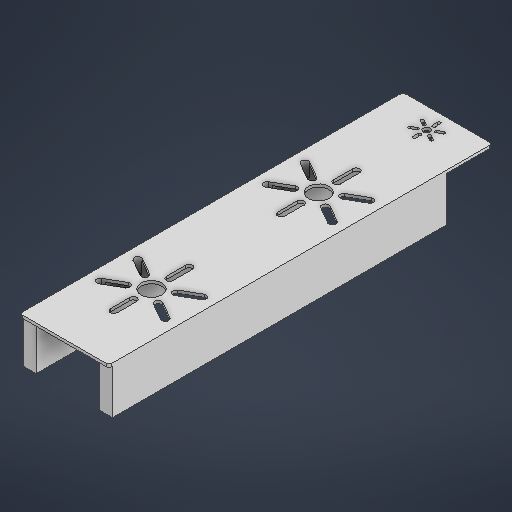
# Autodesk Inventor part: top
Saved by Autodesk Inventor 2027 (Build 310192060, 192F)
## iProperties
Created: 2026-08-21
Part Number: top
Material: Ogólny
Document SubType Name: Modeling
Designer: User
Density: 1 g/cm^3
Appearance: Domyślna
Author: User
Autodesk Inventor part; units mm, degrees
ref_plane "YZ Plane" through (0, 0, 0) normal (1, 0, 0) x (0, 1, 0)
ref_plane "XZ Plane" through (0, 0, 0) normal (0, 1, 0) x (-1, 0, 0)
ref_plane "XY Plane" through (0, 0, 0) normal (0, 0, 1) x (1, 0, 0)
sketch "Szkic1" plane through (0, 0, 0) normal (0, 1, 0) x (-1, 0, 0)
  line L0 (22.75, 95) -> (-22.75, 95)
  line L1 (-22.75, 95) -> (-22.75, -95)
  line L2 (-22.75, -95) -> (22.75, -95)
  line L3 (22.75, -95) -> (22.75, 95)
  line L4 (22.75, 95) -> (-22.75, -95) construction
  line L5 (-22.75, 95) -> (22.75, -95) construction
  line L6 (-32, -97.5) -> (32, -97.5)
  line L7 (32, -97.5) -> (32, 97.5)
  line L8 (32, 97.5) -> (-32, 97.5)
  line L9 (-32, 97.5) -> (-32, -97.5)
  line L10 (-32, -97.5) -> (32, 97.5) construction
  line L11 (32, -97.5) -> (-32, 97.5) construction
  line L12 (32, 97.5) -> (-32, 97.5)
  line L13 (-32, 97.5) -> (-32, 147.5)
  line L14 (-32, 147.5) -> (32, 147.5)
  line L15 (32, 147.5) -> (32, 97.5)
  line L16 (22.75, -95) -> (22.75, -97.5)
  line L17 (-22.75, -95) -> (-22.75, -97.5)
  line L18 (22.75, 95) -> (22.75, 145)
  line L19 (22.75, 145) -> (-22.75, 145)
  line L20 (-22.75, 145) -> (-22.75, 95)
  line L21 (22.75, 145) -> (22.75, 147.5)
  line L22 (-22.75, 145) -> (-22.75, 147.5)
  line L23 (22.75, -95) -> (32, -95)
  line L24 (-22.75, -95) -> (-32, -95)
  line L25 (22.75, 145) -> (32, 145)
  line L26 (-22.75, 145) -> (-32, 145)
  point P0 (0, 0)
  point P1 (0, 0)
  dimension "d0" = 45.5
  dimension "d1" = 190
  dimension "d2" = 64
  dimension "d3" = 195
  dimension "d4" = 50
  dimension "d5" = 50
  dimension "d6" = 0
  dimension "d7" = 0
  constraints: 54 end point, 12 perpendicular, 10 point on line, 6 parallel, 4 midpoint, 2 collinear, 2 horizontal
  measures "d0" distance of L2.end L1.end
  measures "d1" distance of L1.end L0.end
  measures "d2" distance of L9.start L7.end
  measures "d3" distance of L7.end L7.start
  measures "d4" distance of L9.start L14.start
  measures "d5" distance of L0.start L18.end
  measures "d6" distance of point (0, 0) point (0, 0)
  measures "d7" distance of point (0, 0) point (0, 0)
extrude "Wyciągnięcie proste1" add sketch "Szkic1" along normal blind 2
extrude "Wyciągnięcie proste2" add sketch "Szkic1" against normal blind 32 contours L18 L8 L7 L23 L3 | L1 L24 L9 L8 L20 | L18 L25 L15 L8 | L8 L13 L26 L20
sketch "Szkic2" plane through (0, -32, 0) normal (0, -1, 0) x (1, 0, 0)
  line L0 (32, 147.5) -> (-32, 147.5)
  line L1 (-32, -97.5) -> (32, -97.5)
  line L2 (-32, 147.5) -> (32, 147.5)
  line L3 (32, 147.5) -> (32, -97.5)
  line L4 (32, -97.5) -> (-32, -97.5)
  line L5 (-32, -97.5) -> (-32, 147.5)
  line L6 (-32, 147.5) -> (32, 147.5)
  line L7 (0, 147.5) -> (0, -97.5) construction
  line L8 (32, 145) -> (32, -95)
  line L9 (32, -97.5) -> (32, 145)
  line L10 (32, 145) -> (32, 23.75)
  line L11 (32, 23.75) -> (-32, 23.75) construction
  line L12 (22.75, 97.5) -> (22.75, 145)
  line L13 (22.75, 145) -> (22.75, -97.5)
  line L14 (22.75, 23.75) -> (32, 23.75) construction
  line L15 (22.75, 145) -> (22.75, 147.5) construction
  line L16 (22.75, 147.5) -> (32, 147.5) construction
  line L17 (27.375, 147.5) -> (27.375, 23.75) construction
  line L18 (27.375, 147.5) -> (27.375, 137.5) construction
  circle A0 centre (27.375, 137.5) radius 2.4
  circle A1 centre (27.375, 137.5) radius 1
  circle A2 centre (-27.375, 137.5) radius 1
  circle A3 centre (-27.375, 137.5) radius 2.4
  circle A4 centre (-27.375, -90) radius 2.4
  circle A5 centre (-27.375, -90) radius 1
  circle A6 centre (27.375, -90) radius 1
  circle A7 centre (27.375, -90) radius 2.4
  line L19 (-32, -97.5) -> (-32, 147.5) projected
  line L20 (-32, 147.5) -> (32, 147.5)
  point P0 (0, 0)
  point P1 (0, 0)
  dimension "d12" = 10
  dimension "d13" = 4.8
  dimension "d14" = 2
  constraints: 40 end point, 8 centre point, 6 midpoint, 6 symmetric about line, 5 coincident, 4 point on line, 3 collinear, 3 parallel, 3 perpendicular, 1 horizontal, 1 vertical, 6 other
  measures "d12" distance of L17.start L18.end
  measures "d13" diameter of A0
  measures "d14" diameter of A1
extrude "Wyciągnięcie proste3" cut sketch "Szkic2" against normal blind 10 contours A0 | A1 | A2 | A3 | A4 | A5 | A6 | A7
fillet "Zaokrąglenie1" radius 2 2 edges at (32, 1, 147.5) (-32, 1, 147.5)
sketch "Szkic3" plane through (0, 2, 0) normal (0, 1, 0) x (1, 0, 0)
  line L0 (32, 97.5) -> (-32, 97.5) projected
  line L1 (-30, -147.5) -> (30, -147.5) projected
  line L2 (-30, 97.5) -> (30, 97.5)
  line L3 (30, 97.5) -> (30, -147.5)
  line L4 (30, -147.5) -> (-30, -147.5)
  line L5 (-30, -147.5) -> (-30, 97.5)
  line L6 (0, 97.5) -> (0, -147.5) construction
  line L7 (-30, -25) -> (30, -25) construction
  line L8 (0, -25) -> (0, 95) construction
  circle A0 centre (0, 35) radius 7.5
  line L9 (0, 35) -> (0, 55) construction
  line L10 (0, 62) -> (0, 48) construction
  line L11 (-2.5, 62) -> (-2.5, 48)
  line L12 (2.5, 48) -> (2.5, 62)
  arc A1 (2.5, 62) -> (-2.5, 62) centre (0, 62) ccw
  arc A2 (-2.5, 48) -> (2.5, 48) centre (0, 48) ccw
  arc A3 (-12.5083, 39.3349) -> (-10.0083, 43.6651) centre (-11.2583, 41.5) ccw
  line L13 (0, 35) -> (-17.3205, 45) construction
  line L14 (51.9615, 5) -> (-51.9615, 65) construction
  line L15 (-23.3827, 48.5) -> (-11.2583, 41.5) construction
  line L16 (-24.6327, 46.3349) -> (-12.5083, 39.3349)
  line L17 (-10.0083, 43.6651) -> (-22.1327, 50.6651)
  arc A4 (-22.1327, 50.6651) -> (-24.6327, 46.3349) centre (-23.3827, 48.5) ccw
  arc A5 (-10.0083, 26.3349) -> (-12.5083, 30.6651) centre (-11.2583, 28.5) ccw
  line L18 (0, 35) -> (-17.3205, 25) construction
  line L19 (51.9615, 65) -> (-51.9615, 5) construction
  line L20 (-23.3827, 21.5) -> (-11.2583, 28.5) construction
  line L21 (-22.1327, 19.3349) -> (-10.0083, 26.3349)
  line L22 (-12.5083, 30.6651) -> (-24.6327, 23.6651)
  arc A6 (-24.6327, 23.6651) -> (-22.1327, 19.3349) centre (-23.3827, 21.5) ccw
  arc A7 (2.5, 22) -> (-2.5, 22) centre (0, 22) ccw
  line L23 (0, 35) -> (0, 15) construction
  line L24 (0, 95) -> (0, -25) construction
  line L25 (0, 8) -> (0, 22) construction
  line L26 (2.5, 8) -> (2.5, 22)
  line L27 (-2.5, 22) -> (-2.5, 8)
  arc A8 (-2.5, 8) -> (2.5, 8) centre (0, 8) ccw
  arc A9 (12.5083, 30.6651) -> (10.0083, 26.3349) centre (11.2583, 28.5) ccw
  line L28 (0, 35) -> (17.3205, 25) construction
  line L29 (-51.9615, 65) -> (51.9615, 5) construction
  line L30 (23.3827, 21.5) -> (11.2583, 28.5) construction
  line L31 (24.6327, 23.6651) -> (12.5083, 30.6651)
  line L32 (10.0083, 26.3349) -> (22.1327, 19.3349)
  arc A10 (22.1327, 19.3349) -> (24.6327, 23.6651) centre (23.3827, 21.5) ccw
  arc A11 (10.0083, 43.6651) -> (12.5083, 39.3349) centre (11.2583, 41.5) ccw
  line L33 (0, 35) -> (17.3205, 45) construction
  line L34 (-51.9615, 5) -> (51.9615, 65) construction
  line L35 (23.3827, 48.5) -> (11.2583, 41.5) construction
  line L36 (22.1327, 50.6651) -> (10.0083, 43.6651)
  line L37 (12.5083, 39.3349) -> (24.6327, 46.3349)
  arc A12 (24.6327, 46.3349) -> (22.1327, 50.6651) centre (23.3827, 48.5) ccw
  line L38 (0, -147.5) -> (0, 97.5) construction
  line L39 (0, -25) -> (0, -145) construction
  circle A13 centre (0, -85) radius 7.5
  line L40 (0, -85) -> (0, -105) construction
  line L41 (0, -112) -> (0, -98) construction
  line L42 (-2.5, -112) -> (-2.5, -98)
  line L43 (2.5, -98) -> (2.5, -112)
  arc A14 (-2.5, -112) -> (2.5, -112) centre (0, -112) ccw
  arc A15 (2.5, -98) -> (-2.5, -98) centre (0, -98) ccw
  arc A16 (-10.0083, -93.6651) -> (-12.5083, -89.3349) centre (-11.2583, -91.5) ccw
  line L44 (0, -85) -> (-17.3205, -95) construction
  line L45 (51.9615, -55) -> (-51.9615, -115) construction
  line L46 (-23.3827, -98.5) -> (-11.2583, -91.5) construction
  line L47 (-24.6327, -96.3349) -> (-12.5083, -89.3349)
  line L48 (-10.0083, -93.6651) -> (-22.1327, -100.6651)
  arc A17 (-24.6327, -96.3349) -> (-22.1327, -100.6651) centre (-23.3827, -98.5) ccw
  arc A18 (-12.5083, -80.6651) -> (-10.0083, -76.3349) centre (-11.2583, -78.5) ccw
  line L49 (0, -85) -> (-17.3205, -75) construction
  line L50 (51.9615, -115) -> (-51.9615, -55) construction
  line L51 (-23.3827, -71.5) -> (-11.2583, -78.5) construction
  line L52 (-22.1327, -69.3349) -> (-10.0083, -76.3349)
  line L53 (-12.5083, -80.6651) -> (-24.6327, -73.6651)
  arc A19 (-22.1327, -69.3349) -> (-24.6327, -73.6651) centre (-23.3827, -71.5) ccw
  arc A20 (-2.5, -72) -> (2.5, -72) centre (0, -72) ccw
  line L54 (0, -85) -> (0, -65) construction
  line L55 (0, -145) -> (0, -25) construction
  line L56 (0, -58) -> (0, -72) construction
  line L57 (2.5, -58) -> (2.5, -72)
  line L58 (-2.5, -72) -> (-2.5, -58)
  arc A21 (2.5, -58) -> (-2.5, -58) centre (0, -58) ccw
  arc A22 (10.0083, -76.3349) -> (12.5083, -80.6651) centre (11.2583, -78.5) ccw
  line L59 (0, -85) -> (17.3205, -75) construction
  line L60 (-51.9615, -115) -> (51.9615, -55) construction
  line L61 (23.3827, -71.5) -> (11.2583, -78.5) construction
  line L62 (24.6327, -73.6651) -> (12.5083, -80.6651)
  line L63 (10.0083, -76.3349) -> (22.1327, -69.3349)
  arc A23 (24.6327, -73.6651) -> (22.1327, -69.3349) centre (23.3827, -71.5) ccw
  arc A24 (12.5083, -89.3349) -> (10.0083, -93.6651) centre (11.2583, -91.5) ccw
  line L64 (0, -85) -> (17.3205, -95) construction
  line L65 (-51.9615, -55) -> (51.9615, -115) construction
  line L66 (23.3827, -98.5) -> (11.2583, -91.5) construction
  line L67 (22.1327, -100.6651) -> (10.0083, -93.6651)
  line L68 (12.5083, -89.3349) -> (24.6327, -96.3349)
  arc A25 (22.1327, -100.6651) -> (24.6327, -96.3349) centre (23.3827, -98.5) ccw
  point P0 (0, 0)
  point P1 (30, 97.5)
  point P2 (0, 97.5)
  dimension "d18" = 15
  dimension "d19" = 62.5
  dimension "d20" = 20
  dimension "d21" = 7
  dimension "d22" = 5
  dimension "d25" = 360
  constraints: 158 end point, 60 symmetric about line, 48 point on circle, 26 centre point, 26 point on line, 8 midpoint, 4 tangent, 3 parallel, 2 coincident, 1 horizontal, 1 perpendicular, 114 other
  measures "d18" diameter of A0
  measures "d19" distance of point (0, 97.5) L9.start
  measures "d20" distance of L9.start L9.end
  measures "d21" distance of L9.end L10.end
  measures "d22" diameter of A2
extrude "Wyciągnięcie proste4" cut sketch "Szkic3" against normal blind 10 contours A0 | A1 L12 A2 L11 | L16 A4 L17 A3 | L21 A6 L22 A5 | L26 A8 L27 A7 | L31 A10 L32 A9 | L36 A12 L37 A11 | A13 | L42 A15 L43 A14 | L48 A17 L47 A16 | L53 A19 L52 A18 | L58 A21 L57 A20 | L63 A23 L62 A22 | L68 A25 L67 A24
move faces "Przesuń1" translate (0, 0, -30) faces at (10.6667, 0.6667, -97.5)
fillet "Zaokrąglenie2" radius 2 2 edges at (32, 1, -127.5) (-32, 1, -127.5)
sketch "Szkic4" plane through (0, 2, 0) normal (0, 1, 0) x (1, 0, 0)
  line L0 (30, 127.5) -> (-30, 127.5) projected
  circle A0 centre (0, 112.5) radius 2.5
  line L1 (0, 112.5) -> (0, 105.5)
  line L2 (0, 103.5) -> (0, 107.5) construction
  line L3 (1, 103.5) -> (1, 107.5)
  line L4 (-1, 107.5) -> (-1, 103.5)
  arc A1 (-1, 103.5) -> (1, 103.5) centre (0, 103.5) ccw
  arc A2 (1, 107.5) -> (-1, 107.5) centre (0, 107.5) ccw
  line L5 (0, 112.5) -> (6.0622, 109)
  line L6 (7.7942, 108) -> (4.3301, 110) construction
  line L7 (8.2942, 108.866) -> (4.8301, 110.866)
  line L8 (3.8301, 109.134) -> (7.2942, 107.134)
  arc A3 (7.2942, 107.134) -> (8.2942, 108.866) centre (7.7942, 108) ccw
  arc A4 (4.8301, 110.866) -> (3.8301, 109.134) centre (4.3301, 110) ccw
  line L9 (0, 112.5) -> (6.0622, 116)
  line L10 (7.7942, 117) -> (4.3301, 115) construction
  line L11 (7.2942, 117.866) -> (3.8301, 115.866)
  line L12 (4.8301, 114.134) -> (8.2942, 116.134)
  arc A5 (8.2942, 116.134) -> (7.2942, 117.866) centre (7.7942, 117) ccw
  arc A6 (3.8301, 115.866) -> (4.8301, 114.134) centre (4.3301, 115) ccw
  line L13 (0, 112.5) -> (0, 119.5)
  line L14 (0, 121.5) -> (0, 117.5) construction
  line L15 (-1, 121.5) -> (-1, 117.5)
  line L16 (1, 117.5) -> (1, 121.5)
  arc A7 (1, 121.5) -> (-1, 121.5) centre (0, 121.5) ccw
  arc A8 (-1, 117.5) -> (1, 117.5) centre (0, 117.5) ccw
  line L17 (0, 112.5) -> (-6.0622, 116)
  line L18 (-7.7942, 117) -> (-4.3301, 115) construction
  line L19 (-8.2942, 116.134) -> (-4.8301, 114.134)
  line L20 (-3.8301, 115.866) -> (-7.2942, 117.866)
  arc A9 (-7.2942, 117.866) -> (-8.2942, 116.134) centre (-7.7942, 117) ccw
  arc A10 (-4.8301, 114.134) -> (-3.8301, 115.866) centre (-4.3301, 115) ccw
  line L21 (0, 112.5) -> (-6.0622, 109)
  line L22 (-7.7942, 108) -> (-4.3301, 110) construction
  line L23 (-7.2942, 107.134) -> (-3.8301, 109.134)
  line L24 (-4.8301, 110.866) -> (-8.2942, 108.866)
  arc A11 (-8.2942, 108.866) -> (-7.2942, 107.134) centre (-7.7942, 108) ccw
  arc A12 (-3.8301, 109.134) -> (-4.8301, 110.866) centre (-4.3301, 110) ccw
  point P0 (0, 0)
  point P1 (0, 127.5)
  dimension "d34" = 5
  dimension "d36" = 2
  dimension "d37" = 2
  dimension "d40" = 360
  dimension "d43" = 15
  dimension "d44" = 5
  constraints: 60 end point, 24 point on circle, 13 centre point, 6 point on line, 4 tangent, 2 coincident, 2 midpoint, 1 parallel, 83 other
  measures "d34" diameter of A0
  measures "d36" distance of L1.end L2.end
  measures "d37" diameter of A2
  measures "d43" distance of point (0, 127.5) L1.start
  measures "d44" distance of L2.end L1.start
extrude "Wyciągnięcie proste5" cut sketch "Szkic4" against normal blind 10
